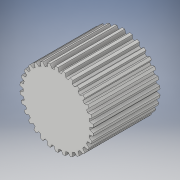
# Autodesk Inventor part: Gear_SBail
Saved by Autodesk Inventor 2019 (Build 230136000, 136)
## iProperties
Created: 2019-04-10
Part Number: Gear_SBail
Material: Generic
Document SubType Name: Modeling
Designer: samson.bailor
Density: 1 g/cm^3
Appearance: Default
Author: samson.bailor
Autodesk Inventor part; units mm, degrees
ref_plane "YZ Plane" through (0, 0, 0) normal (1, 0, 0) x (0, 1, 0)
ref_plane "XZ Plane" through (0, 0, 0) normal (0, 1, 0) x (-1, 0, 0)
ref_plane "XY Plane" through (0, 0, 0) normal (0, 0, 1) x (1, 0, 0)
sketch "Sketch1" plane through (0, 0, 0) normal (0, 0, 1) x (1, 0, 0)
  line L0 (0, 13.97) -> (0.254, 13.97)
  line L1 (0.254, 13.97) -> (0.508, 13.97)
  line L2 (0, 13.97) -> (-0.508, 13.97)
  line L3 (0.508, 13.97) -> (0.856, 12.6711)
  line L4 (0.508, 13.97) -> (2.6906, 13.97) construction
  line L5 (-0.508, 13.97) -> (2.5555, 13.97) construction
  line L6 (-0.508, 13.97) -> (1.6746, 13.97) construction
  line L7 (-0.508, 13.97) -> (-0.856, 12.6711)
  line L8 (-0.508, 13.97) -> (0.8367, 13.97) construction
  line L9 (-2.4076, 13.7703) -> (-1.7971, 12.5722)
  line L10 (-3.4014, 13.5591) -> (-3.4718, 12.2162)
  line L11 (-2.9045, 13.6647) -> (-2.6561, 13.7175)
  line L12 (-2.6561, 13.7175) -> (-2.4076, 13.7703)
  line L13 (-2.9045, 13.6647) -> (-3.4014, 13.5591)
  line L14 (-5.218, 12.9689) -> (-4.3718, 11.9238)
  line L15 (-6.1462, 12.5556) -> (-5.9358, 11.2275)
  line L16 (-5.6821, 12.7622) -> (-5.4501, 12.8655)
  line L17 (-5.4501, 12.8655) -> (-5.218, 12.9689)
  line L18 (-5.6821, 12.7622) -> (-6.1462, 12.5556)
  line L19 (-7.8004, 11.6006) -> (-6.7553, 10.7543)
  line L20 (-8.6223, 11.0034) -> (-8.1404, 9.748)
  line L21 (-8.2114, 11.302) -> (-8.0059, 11.4513)
  line L22 (-8.0059, 11.4513) -> (-7.8004, 11.6006)
  line L23 (-8.2114, 11.302) -> (-8.6223, 11.0034)
  line L24 (-10.0418, 9.7253) -> (-8.8437, 9.1148)
  line L25 (-10.7217, 8.9702) -> (-9.9893, 7.8425)
  line L26 (-10.3817, 9.3478) -> (-10.2118, 9.5365)
  line L27 (-10.2118, 9.5365) -> (-10.0418, 9.7253)
  line L28 (-10.3817, 9.3478) -> (-10.7217, 8.9702)
  line L29 (-11.8444, 7.4249) -> (-10.5455, 7.0769)
  line L30 (-12.3524, 6.5451) -> (-11.4015, 5.5942)
  line L31 (-12.0984, 6.985) -> (-11.9714, 7.205)
  line L32 (-11.9714, 7.205) -> (-11.8444, 7.4249)
  line L33 (-12.0984, 6.985) -> (-12.3524, 6.5451)
  line L34 (-13.1293, 4.8001) -> (-11.7864, 4.7297)
  line L35 (-13.4432, 3.8338) -> (-12.3155, 3.1015)
  line L36 (-13.2863, 4.317) -> (-13.2078, 4.5585)
  line L37 (-13.2078, 4.5585) -> (-13.1293, 4.8001)
  line L38 (-13.2863, 4.317) -> (-13.4432, 3.8338)
  line L39 (-13.8404, 1.9655) -> (-12.5122, 2.1758)
  line L40 (-13.9466, 0.955) -> (-12.6912, 0.4731)
  line L41 (-13.8935, 1.4603) -> (-13.8669, 1.7129)
  line L42 (-13.8669, 1.7129) -> (-13.8404, 1.9655)
  line L43 (-13.8935, 1.4603) -> (-13.9466, 0.955)
  line L44 (-13.9466, -0.955) -> (-12.6912, -0.4731)
  line L45 (-13.8404, -1.9655) -> (-12.5122, -2.1758)
  line L46 (-13.8935, -1.4603) -> (-13.92, -1.2077)
  line L47 (-13.92, -1.2077) -> (-13.9466, -0.955)
  line L48 (-13.8935, -1.4603) -> (-13.8404, -1.9655)
  line L49 (-13.4432, -3.8338) -> (-12.3155, -3.1015)
  line L50 (-13.1293, -4.8001) -> (-11.7864, -4.7297)
  line L51 (-13.2863, -4.317) -> (-13.3647, -4.0754)
  line L52 (-13.3647, -4.0754) -> (-13.4432, -3.8338)
  line L53 (-13.2863, -4.317) -> (-13.1293, -4.8001)
  line L54 (-12.3524, -6.5451) -> (-11.4015, -5.5942)
  line L55 (-11.8444, -7.4249) -> (-10.5455, -7.0769)
  line L56 (-12.0984, -6.985) -> (-12.2254, -6.765)
  line L57 (-12.2254, -6.765) -> (-12.3524, -6.5451)
  line L58 (-12.0984, -6.985) -> (-11.8444, -7.4249)
  line L59 (-10.7217, -8.9702) -> (-9.9893, -7.8425)
  line L60 (-10.0418, -9.7253) -> (-8.8437, -9.1148)
  line L61 (-10.3817, -9.3478) -> (-10.5517, -9.159)
  line L62 (-10.5517, -9.159) -> (-10.7217, -8.9702)
  line L63 (-10.3817, -9.3478) -> (-10.0418, -9.7253)
  line L64 (-8.6223, -11.0034) -> (-8.1404, -9.748)
  line L65 (-7.8004, -11.6006) -> (-6.7553, -10.7543)
  line L66 (-8.2114, -11.302) -> (-8.4169, -11.1527)
  line L67 (-8.4169, -11.1527) -> (-8.6223, -11.0034)
  line L68 (-8.2114, -11.302) -> (-7.8004, -11.6006)
  line L69 (-6.1462, -12.5556) -> (-5.9358, -11.2275)
  line L70 (-5.218, -12.9689) -> (-4.3718, -11.9238)
  line L71 (-5.6821, -12.7622) -> (-5.9142, -12.6589)
  line L72 (-5.9142, -12.6589) -> (-6.1462, -12.5556)
  line L73 (-5.6821, -12.7622) -> (-5.218, -12.9689)
  line L74 (-3.4014, -13.5591) -> (-3.4718, -12.2162)
  line L75 (-2.4076, -13.7703) -> (-1.7971, -12.5722)
  line L76 (-2.9045, -13.6647) -> (-3.153, -13.6119)
  line L77 (-3.153, -13.6119) -> (-3.4014, -13.5591)
  line L78 (-2.9045, -13.6647) -> (-2.4076, -13.7703)
  line L79 (-0.508, -13.97) -> (-0.856, -12.6711)
  line L80 (0.508, -13.97) -> (0.856, -12.6711)
  line L81 (0, -13.97) -> (-0.254, -13.97)
  line L82 (-0.254, -13.97) -> (-0.508, -13.97)
  line L83 (0, -13.97) -> (0.508, -13.97)
  line L84 (2.4076, -13.7703) -> (1.7971, -12.5722)
  line L85 (3.4014, -13.5591) -> (3.4718, -12.2162)
  line L86 (2.9045, -13.6647) -> (2.6561, -13.7175)
  line L87 (2.6561, -13.7175) -> (2.4076, -13.7703)
  line L88 (2.9045, -13.6647) -> (3.4014, -13.5591)
  line L89 (5.218, -12.9689) -> (4.3718, -11.9238)
  line L90 (6.1462, -12.5556) -> (5.9358, -11.2275)
  line L91 (5.6821, -12.7622) -> (5.4501, -12.8655)
  line L92 (5.4501, -12.8655) -> (5.218, -12.9689)
  line L93 (5.6821, -12.7622) -> (6.1462, -12.5556)
  line L94 (7.8004, -11.6006) -> (6.7553, -10.7543)
  line L95 (8.6223, -11.0034) -> (8.1404, -9.748)
  line L96 (8.2114, -11.302) -> (8.0059, -11.4513)
  line L97 (8.0059, -11.4513) -> (7.8004, -11.6006)
  line L98 (8.2114, -11.302) -> (8.6223, -11.0034)
  line L99 (10.0418, -9.7253) -> (8.8437, -9.1148)
  line L100 (10.7217, -8.9702) -> (9.9893, -7.8425)
  line L101 (10.3817, -9.3478) -> (10.2118, -9.5365)
  line L102 (10.2118, -9.5365) -> (10.0418, -9.7253)
  line L103 (10.3817, -9.3478) -> (10.7217, -8.9702)
  line L104 (11.8444, -7.4249) -> (10.5455, -7.0769)
  line L105 (12.3524, -6.5451) -> (11.4015, -5.5942)
  line L106 (12.0984, -6.985) -> (11.9714, -7.205)
  line L107 (11.9714, -7.205) -> (11.8444, -7.4249)
  line L108 (12.0984, -6.985) -> (12.3524, -6.5451)
  line L109 (13.1293, -4.8001) -> (11.7864, -4.7297)
  line L110 (13.4432, -3.8338) -> (12.3155, -3.1015)
  line L111 (13.2863, -4.317) -> (13.2078, -4.5585)
  line L112 (13.2078, -4.5585) -> (13.1293, -4.8001)
  line L113 (13.2863, -4.317) -> (13.4432, -3.8338)
  line L114 (13.8404, -1.9655) -> (12.5122, -2.1758)
  line L115 (13.9466, -0.955) -> (12.6912, -0.4731)
  line L116 (13.8935, -1.4603) -> (13.8669, -1.7129)
  line L117 (13.8669, -1.7129) -> (13.8404, -1.9655)
  line L118 (13.8935, -1.4603) -> (13.9466, -0.955)
  line L119 (13.9466, 0.955) -> (12.6912, 0.4731)
  line L120 (13.8404, 1.9655) -> (12.5122, 2.1758)
  line L121 (13.8935, 1.4603) -> (13.92, 1.2077)
  line L122 (13.92, 1.2077) -> (13.9466, 0.955)
  line L123 (13.8935, 1.4603) -> (13.8404, 1.9655)
  line L124 (13.4432, 3.8338) -> (12.3155, 3.1015)
  line L125 (13.1293, 4.8001) -> (11.7864, 4.7297)
  line L126 (13.2863, 4.317) -> (13.3647, 4.0754)
  line L127 (13.3647, 4.0754) -> (13.4432, 3.8338)
  line L128 (13.2863, 4.317) -> (13.1293, 4.8001)
  line L129 (12.3524, 6.5451) -> (11.4015, 5.5942)
  line L130 (11.8444, 7.4249) -> (10.5455, 7.0769)
  line L131 (12.0984, 6.985) -> (12.2254, 6.765)
  line L132 (12.2254, 6.765) -> (12.3524, 6.5451)
  line L133 (12.0984, 6.985) -> (11.8444, 7.4249)
  line L134 (10.7217, 8.9702) -> (9.9893, 7.8425)
  line L135 (10.0418, 9.7253) -> (8.8437, 9.1148)
  line L136 (10.3817, 9.3478) -> (10.5517, 9.159)
  line L137 (10.5517, 9.159) -> (10.7217, 8.9702)
  line L138 (10.3817, 9.3478) -> (10.0418, 9.7253)
  line L139 (8.6223, 11.0034) -> (8.1404, 9.748)
  line L140 (7.8004, 11.6006) -> (6.7553, 10.7543)
  line L141 (8.2114, 11.302) -> (8.4169, 11.1527)
  line L142 (8.4169, 11.1527) -> (8.6223, 11.0034)
  line L143 (8.2114, 11.302) -> (7.8004, 11.6006)
  line L144 (6.1462, 12.5556) -> (5.9358, 11.2275)
  line L145 (5.218, 12.9689) -> (4.3718, 11.9238)
  line L146 (5.6821, 12.7622) -> (5.9142, 12.6589)
  line L147 (5.9142, 12.6589) -> (6.1462, 12.5556)
  line L148 (5.6821, 12.7622) -> (5.218, 12.9689)
  line L149 (3.4014, 13.5591) -> (3.4718, 12.2162)
  line L150 (2.4076, 13.7703) -> (1.7971, 12.5722)
  line L151 (2.9045, 13.6647) -> (3.153, 13.6119)
  line L152 (3.153, 13.6119) -> (3.4014, 13.5591)
  line L153 (2.9045, 13.6647) -> (2.4076, 13.7703)
  arc A0 (-8.1404, 9.748) -> (-8.8437, 9.1148) centre (0, 0) ccw
  arc A1 (-5.9358, 11.2275) -> (-6.7553, 10.7543) centre (0, 0) ccw
  arc A2 (-3.4718, 12.2162) -> (-4.3718, 11.9238) centre (0, 0) ccw
  arc A3 (-0.856, 12.6711) -> (-1.7971, 12.5722) centre (0, 0) ccw
  arc A4 (1.7971, 12.5722) -> (0.856, 12.6711) centre (0, 0) ccw
  arc A5 (4.3718, 11.9238) -> (3.4718, 12.2162) centre (0, 0) ccw
  arc A6 (6.7553, 10.7543) -> (5.9358, 11.2275) centre (0, 0) ccw
  arc A7 (8.8437, 9.1148) -> (8.1404, 9.748) centre (0, 0) ccw
  arc A8 (10.5455, 7.0769) -> (9.9893, 7.8425) centre (0, 0) ccw
  arc A9 (11.7864, 4.7297) -> (11.4015, 5.5942) centre (0, 0) ccw
  arc A10 (12.5122, 2.1758) -> (12.3155, 3.1015) centre (0, 0) ccw
  arc A11 (12.6912, -0.4731) -> (12.6912, 0.4731) centre (0, 0) ccw
  arc A12 (12.3155, -3.1015) -> (12.5122, -2.1758) centre (0, 0) ccw
  arc A13 (11.4015, -5.5942) -> (11.7864, -4.7297) centre (0, 0) ccw
  arc A14 (9.9893, -7.8425) -> (10.5455, -7.0769) centre (0, 0) ccw
  arc A15 (8.1404, -9.748) -> (8.8437, -9.1148) centre (0, 0) ccw
  arc A16 (5.9358, -11.2275) -> (6.7553, -10.7543) centre (0, 0) ccw
  arc A17 (3.4718, -12.2162) -> (4.3718, -11.9238) centre (0, 0) ccw
  arc A18 (0.856, -12.6711) -> (1.7971, -12.5722) centre (0, 0) ccw
  arc A19 (-1.7971, -12.5722) -> (-0.856, -12.6711) centre (0, 0) ccw
  arc A20 (-4.3718, -11.9238) -> (-3.4718, -12.2162) centre (0, 0) ccw
  arc A21 (-6.7553, -10.7543) -> (-5.9358, -11.2275) centre (0, 0) ccw
  arc A22 (-8.8437, -9.1148) -> (-8.1404, -9.748) centre (0, 0) ccw
  arc A23 (-10.5455, -7.0769) -> (-9.9893, -7.8425) centre (0, 0) ccw
  arc A24 (-11.7864, -4.7297) -> (-11.4015, -5.5942) centre (0, 0) ccw
  arc A25 (-12.5122, -2.1758) -> (-12.3155, -3.1015) centre (0, 0) ccw
  arc A26 (-12.6912, 0.4731) -> (-12.6912, -0.4731) centre (0, 0) ccw
  arc A27 (-12.3155, 3.1015) -> (-12.5122, 2.1758) centre (0, 0) ccw
  arc A28 (-9.9893, 7.8425) -> (-10.5455, 7.0769) centre (0, 0) ccw
  arc A29 (-11.4015, 5.5942) -> (-11.7864, 4.7297) centre (0, 0) ccw
  dimension "d4" = 0.254
  dimension "d5" = 0.254
  dimension "d7" = 0.508
  dimension "d9" = 75
  dimension "d12" = 105
  dimension "d15" = 360
  constraints: 308 end point, 150 equal length, 30 point on line, 5 horizontal, 4 vertical alignment, 267 other
  measures "d4" distance of L0.start L0.end
  measures "d5" distance of L0.end L1.end
  measures "d7" distance of L0.start L2.end
  measures "d9" angle of L3 L4
  measures "d12" angle of L7 L8
extrude "Extrusion1" add sketch "Sketch1" along normal blind 25.4
body "Solid1"
